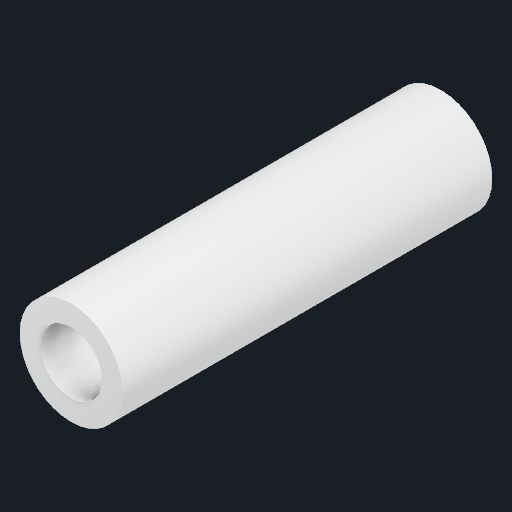
# Autodesk Inventor part: 20x5 mm spacer
Saved by Autodesk Inventor 2024.3 (Build 283343000, 343)
## iProperties
Created: 2024-10-05
Part Number: 20x5 mm spacer
Material: Aluminum 6061
Document SubType Name: Modeling
Designer: MFil
Density: 2.7 g/cm^3
Appearance: Aluminum - Flat
Mass: 0.610726 g
Surface Area: 4.77522 cm^2
Volume: 0.226195 cm^3
Author: MFil
Autodesk Inventor part; units mm, degrees
ref_plane "YZ Plane" through (0, 0, 0) normal (1, 0, 0) x (0, 1, 0)
ref_plane "XZ Plane" through (0, 0, 0) normal (0, 1, 0) x (-1, 0, 0)
ref_plane "XY Plane" through (0, 0, 0) normal (0, 0, 1) x (1, 0, 0)
sketch "Sketch1" plane through (0, 0, 0) normal (0, 0, 1) x (1, 0, 0)
  circle A0 centre (-21.92, 0) radius 1.6 projected
  circle A1 centre (-21.92, 0) radius 2.5
  circle A2 centre (-21.92, 0) radius 1.5
  point P0 (0, 0)
  dimension "d0" = 5
  dimension "d1" = 3
  constraints: 2 centre point, 2 coincident
  measures "d0" diameter of A1
  measures "d1" diameter of A2
extrude "Extrusion1" add sketch "Sketch1" along normal blind 18 contours A0 | A1
body "Solid1"
